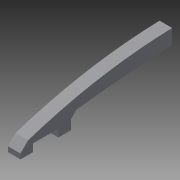
# Autodesk Inventor part: CameraArm
Saved by Autodesk Inventor 2015 (Build 190159000, 159)
## iProperties
Created: 2015-11-25
Part Number: CameraArm
Material: Generic
Document SubType Name: Modeling
Designer: Lauszus
Density: 1 g/cm^3
Appearance: Default
Author: Lauszus
Autodesk Inventor part; units mm, degrees
ref_plane "YZ Plane" through (0, 0, 0) normal (1, 0, 0) x (0, 1, 0)
ref_plane "XZ Plane" through (0, 0, 0) normal (0, 1, 0) x (-1, 0, 0)
ref_plane "XY Plane" through (0, 0, 0) normal (0, 0, 1) x (1, 0, 0)
sketch "Sketch1" plane through (0, 0, 0) normal (0, 0, 1) x (1, 0, 0)
  line L0 (-40, 0) -> (-20, 0)
  line L1 (-20, 0) -> (-20, 5)
  line L2 (-20, 5) -> (-40, 5)
  line L3 (-40, 5) -> (-40, 0)
  arc A0 (20, 15) -> (-37, 5) centre (25.6963, -184.9189) ccw
  arc A1 (20, 9) -> (-25, 5) centre (32.8594, -390.7932) ccw
  line L4 (-37, 5) -> (-25, 5)
  line L5 (20, 15) -> (20, 9)
  line L6 (-20, 5) -> (-20, 5.6987)
  point P0 (0, 0)
  dimension "d0" = 20
  dimension "d9" = 5
  dimension "d11" = 40
  dimension "d13" = 20
  dimension "d14" = 5
  dimension "d16" = 10
  dimension "d17" = 3
  dimension "d19" = 6
  dimension "d20" = 40
  dimension "d21" = 200
  dimension "d22" = 400
  dimension "d24" = 12
  constraints: 14 end point, 5 point on circle, 2 centre point, 2 parallel, 2 point on line, 1 collinear, 1 horizontal, 1 perpendicular, 1 vertical
  measures "d0" distance of L1.end L2.end
  measures "d9" distance of L2.end L0.start
  measures "d11" distance from line of L1 L5.start
  measures "d13" distance from line of point (0, 0) L1
  measures "d14" distance from line of point (0, 0) L2
  measures "d16" vertical distance of L5.start L1.end
  measures "d17" distance from line of L3 L4.start
  measures "d19" distance of L5.end L5.start
  measures "d20" distance from line of L1 L5.end
  measures "d21" radius of A0
  measures "d22" radius of A1
  measures "d24" distance of L4.start L4.end
extrude "Extrusion3" add sketch "Sketch1" along normal blind 5
sketch "Sketch3" plane through (-40, 0, 0) normal (0, -1, 0) x (1, 0, 0)
  line L0 (0, 5) -> (20, 5) projected
  line L1 (5, 5) -> (15, 5)
  line L2 (15, 5) -> (15, 0)
  line L3 (15, 0) -> (5, 0)
  line L4 (5, 0) -> (5, 5)
  line L5 (0, 0) -> (0, 5) projected
  point P0 (40, 0)
  dimension "d27" = 10
  dimension "d28" = 5
  constraints: 8 end point, 2 parallel, 1 horizontal, 1 perpendicular, 1 point on line
  measures "d27" distance of L2.end L3.end
  measures "d28" distance between parallel lines of L5 L4
extrude "Extrusion4" cut sketch "Sketch3" against normal blind 3
chamfer "Chamfer1" distance 2 angle 45 1 edges at (-20, 5.6987, 2.5)
chamfer "Chamfer2" distance 3 angle 45 1 edges at (-40, 5, 2.5)
body "Solid2"
